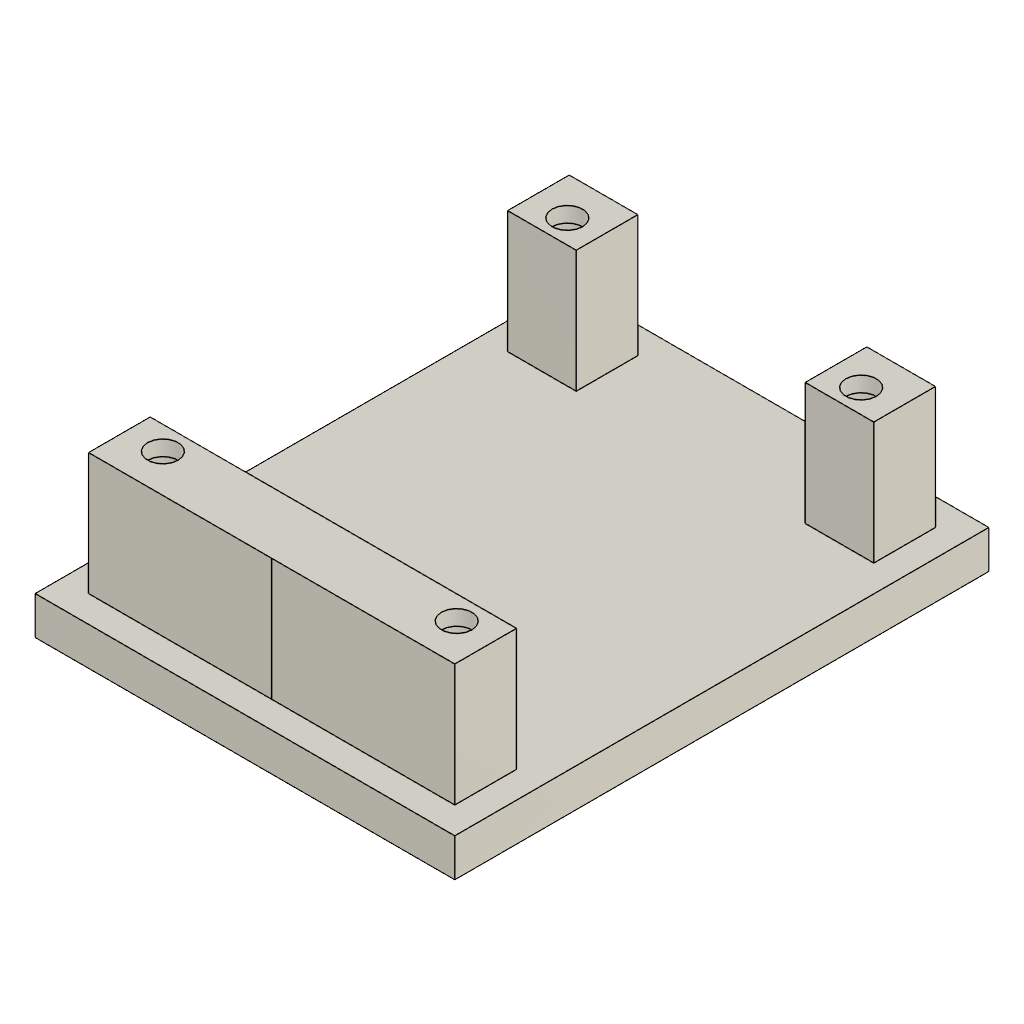
Case assembly (Autodesk Fusion 360 archive; units mm, degrees)
design "Board Case Top"
part number: 2026-09-13-14-46-25-976
Autodesk Fusion 360 part; units mm, degrees
sketch "Sketch1" plane through (0, 0, 0) normal (0, 0, 1) x (1, 0, 0)
  line L0 (25, 33) -> (-25, 33)
  line L1 (-27.5, 35) -> (-27.5, -35)
  line L2 (-25, 33) -> (-25, -33)
  line L3 (27.5, -35) -> (27.5, 35)
  circle A0 centre (19.25, -26.5) radius 2
  line L4 (-19.25, -26.5) -> (19.25, -26.5)
  line L5 (0, 0) -> (0, -26.5)
  circle A1 centre (19.25, 26.5) radius 2
  line L6 (0, 0) -> (0, 26.5)
  line L7 (27.5, 35) -> (-27.5, -35) construction
  circle A2 centre (-19.25, -26.5) radius 2
  line L8 (-25, 33) -> (25, -33) construction
  line L9 (25, 33) -> (-25, -33) construction
  line L10 (27.5, 35) -> (27.5, -35)
  line L11 (27.5, -35) -> (-27.5, -35)
  line L12 (27.5, 35) -> (-27.5, 35)
  line L13 (25, -33) -> (25, 33)
  line L14 (-27.5, -35) -> (-27.5, 35)
  line L15 (27.5, 35) -> (-27.5, 35)
  circle A3 centre (-19.25, 26.5) radius 2
  line L16 (-27.5, -35) -> (27.5, -35)
  line L17 (-27.5, 35) -> (27.5, -35) construction
  line L18 (-27.5, -35) -> (27.5, -35)
  line L19 (0, -35) -> (0, 35)
  line L20 (-19.25, 26.5) -> (19.25, 26.5)
  line L21 (-27.5, 35) -> (27.5, 35)
  line L22 (-25, -33) -> (25, -33)
  dimension "d2" = 70
  dimension "d3" = 55
  dimension "d4" = 55
  dimension "d5" = 26.5
  dimension "d6" = 26.5
  dimension "d7" = 38.5
  dimension "d8" = 38.5
  dimension "d9" = 4
  dimension "d10" = 4
  dimension "d11" = 4
  dimension "d12" = 4
  constraint midpoint L5.start L19
  constraint coincident L5.start L6.start
  constraint vertical L19
  constraint midpoint L19.end L15
  constraint perpendicular L15 L19
  constraint midpoint L19.start L16
  constraint perpendicular L16 L19
  constraint horizontal L21
  constraint vertical L10
  constraint horizontal L11
  constraint vertical L14
  constraint coincident L6.end L19
  constraint parallel L5 L19
  constraint midpoint L6.end L20
  constraint perpendicular L6 L20
  constraint midpoint L5.end L4
  constraint perpendicular L4 L19
  constraint coincident L4.start A2.centre
  constraint coincident A0.centre L4.end
  constraint coincident A1.centre L20.end
  constraint coincident A3.centre L20.start
  constraint horizontal L0
  constraint perpendicular L0 L2
  constraint parallel L0 L22
  constraint parallel L2 L13
  constraint coincident L5.start L9
  constraint coincident L5.start L8
  constraint horizontal L12
  constraint perpendicular L1 L12
  constraint parallel L12 L18
  constraint parallel L1 L3
  constraint coincident L5.start L7
  constraint coincident L5.start L17
  measures "d2" distance of L19.start L19.end
  measures "d3" distance of L3.end L1.start
  measures "d4" distance of L3.start L1.end
  measures "d5" distance of L6.end L5.start
  measures "d6" distance of L5.end L5.start
  measures "d7" distance of A3.centre A1.centre
  measures "d8" distance of A0.centre L4.start
  measures "d9" diameter of A2
  measures "d10" diameter of A0
  measures "d11" diameter of A1
  measures "d12" diameter of A3
extrude "Extrude1" add sketch "Sketch1" along normal blind 5
sketch "Sketch2" plane through (0, 0, 5) normal (0, 0, 1) x (-1, 0, 0)
  circle A0 centre (-19.25, 26.5) radius 2
  circle A1 centre (19.25, -26.5) radius 2
  circle A2 centre (19.25, 26.5) radius 2
  circle A3 centre (-19.25, -26.5) radius 2
  line L0 (27.5, 35) -> (-27.5, 35)
  line L1 (-27.5, 35) -> (-27.5, -35)
  line L2 (-27.5, -35) -> (27.5, -35)
  line L3 (27.5, -35) -> (27.5, 35)
  line L4 (19.25, -26.5) -> (-19.25, -26.5)
  line L5 (19.25, 26.5) -> (-19.25, 26.5)
  line L6 (-27.5, 29.5868) -> (27.5, 29.5868)
  line L7 (27.5, 29.5868) -> (27.5, 23.4132)
  line L8 (27.5, 23.4132) -> (-27.5, 23.4132)
  line L9 (-27.5, 23.4132) -> (-27.5, 29.5868)
  line L10 (-27.5, 29.5868) -> (27.5, 23.4132) construction
  line L11 (27.5, 29.5868) -> (-27.5, 23.4132) construction
  line L12 (-27.5, -29.5868) -> (-27.5, -23.4132)
  line L13 (-27.5, -23.4132) -> (27.5, -23.4132)
  line L14 (27.5, -29.5868) -> (-27.5, -29.5868)
  line L15 (27.5, -23.4132) -> (27.5, -29.5868)
  point P0 (0, 26.5)
  constraint coincident A1.centre L4.start
  constraint coincident A3.centre L4.end
  constraint coincident A2.centre L5.start
  constraint coincident A0.centre L5.end
  constraint horizontal L6
  constraint perpendicular L6 L7
  constraint parallel L6 L8
  constraint parallel L7 L9
  constraint coincident L10 P0
  constraint coincident L11 P0
  constraint coincident L1 L6.start
  constraint midpoint L5 P0
  constraint horizontal L13
  constraint perpendicular L13 L15
  constraint parallel L13 L14
  constraint parallel L12 L15
extrude "Extrude2" add sketch "Sketch2" along normal blind 16 contours L1 L3 L6 L7 L8 L9 | L1 L3 L12 L13 L14 L15
sketch "Sketch3" plane through (0, 0, 5) normal (0, 0, 1) x (-1, 0, 0)
  line L0 (27.5, 23.4132) -> (-27.5, 23.4132)
  line L1 (-27.5, 23.4132) -> (-27.5, -23.4132)
  line L2 (-27.5, -23.4132) -> (27.5, -23.4132)
  line L3 (27.5, -23.4132) -> (27.5, 23.4132)
  line L4 (-25, -32.5) -> (-25, 32.5)
  line L5 (-25, 32.5) -> (25, 32.5)
  line L6 (25, 32.5) -> (25, -32.5)
  line L7 (25, -32.5) -> (-25, -32.5)
  line L8 (25, -32.5) -> (-25, -32.5)
  line L9 (-25, -32.5) -> (-25, -29.5)
  line L10 (-25, -29.5) -> (25, -29.5)
  line L11 (25, -29.5) -> (25, -32.5)
  line L12 (25, 32.5) -> (-25, 32.5)
  line L13 (-25, 32.5) -> (-25, 29)
  line L14 (-25, 29) -> (25, 29)
  line L15 (25, 29) -> (25, 32.5)
  dimension "d17" = 65
  dimension "d18" = 50
  constraint horizontal L5
  constraint perpendicular L5 L6
  constraint parallel L5 L7
  constraint parallel L4 L6
  constraint horizontal L8
  constraint vertical L9
  constraint horizontal L10
  constraint vertical L11
  constraint coincident L4 L9.end
  constraint horizontal L12
  constraint vertical L13
  constraint horizontal L14
  constraint vertical L15
  constraint coincident L4 L13.end
  measures "d17" distance of L6.end L5.end
  measures "d18" distance of L6.end L4.start
extrude "Extrude3" add sketch "Sketch3" along normal blind 16 contours L4 L5 L6 L12 L13 L14 L15 | L4 L6 L7 L8 L9 L10 L11
sketch "Sketch4" plane through (0, 0, 5) normal (0, 0, 1) x (-1, 0, 0)
  line L0 (27.5, 23.4132) -> (-27.5, 23.4132)
  line L1 (-27.5, 23.4132) -> (-27.5, -23.4132)
  line L2 (-27.5, -23.4132) -> (27.5, -23.4132)
  line L3 (27.5, -23.4132) -> (27.5, 23.4132)
  line L4 (-25, -32.5) -> (-25, 32.5)
  line L5 (-25, 32.5) -> (25, 32.5)
  line L6 (25, 32.5) -> (25, -32.5)
  line L7 (25, -32.5) -> (-25, -32.5)
  line L8 (29, 36) -> (-29, 36)
  line L9 (-29, 36) -> (-29, -36)
  line L10 (-29, -36) -> (29, -36)
  line L11 (29, -36) -> (29, 36)
  line L12 (29, 36) -> (-29, -36) construction
  line L13 (-29, 36) -> (29, -36) construction
  dimension "d21" = 65
  dimension "d22" = 50
  constraint horizontal L5
  constraint perpendicular L5 L6
  constraint parallel L5 L7
  constraint parallel L4 L6
  constraint horizontal L8
  constraint perpendicular L8 L9
  constraint parallel L8 L10
  constraint parallel L9 L11
  constraint coincident L12 origin
  constraint coincident L13 origin
  measures "d21" distance of L6.end L5.end
  measures "d22" distance of L6.end L4.start
extrude "Extrude4" cut sketch "Sketch4" along normal blind 20
sketch "Sketch5" plane through (0, 0, 0) normal (0, 0, -1) x (1, 0, 0)
  circle A0 centre (19.25, 26.5) radius 2
  circle A1 centre (-19.25, -26.5) radius 2
  circle A2 centre (-19.25, 26.5) radius 2
  circle A3 centre (19.25, -26.5) radius 2
  line L0 (27.5, 35) -> (-27.5, 35)
  line L1 (-27.5, 35) -> (-27.5, -35)
  line L2 (-27.5, -35) -> (27.5, -35)
  line L3 (27.5, -35) -> (27.5, 35)
  circle A4 centre (19.25, -26.5) radius 3
  circle A5 centre (-19.25, -26.5) radius 3
  circle A6 centre (-19.25, 26.5) radius 3
  circle A7 centre (19.25, 26.5) radius 3
  dimension "d25" = 6
  dimension "d26" = 6
  dimension "d27" = 6
  dimension "d28" = 6
  constraint concentric A3 A4
  measures "d25" diameter of A4
  measures "d26" diameter of A5
  measures "d27" diameter of A6
  measures "d28" diameter of A7
extrude "Extrude5" cut sketch "Sketch5" against normal blind 19 contours A4 | A5 | A6 | A7
sketch "Sketch6" plane through (0, 0, 21) normal (0, 0, 1) x (-1, 0, 0)
  line L0 (-25, -23.4132) -> (-25, -32.5)
  line L1 (-25, -32.5) -> (25, -32.5)
  line L2 (25, -32.5) -> (25, -23.4132)
  line L3 (0, -32.5) -> (0, -31.5)
  line L4 (0, -31.5) -> (25, -31.5)
  line L5 (0, -31.5) -> (-24.1654, -31.5)
  line L6 (-24.1654, -31.5) -> (-25, -31.5)
  line L7 (-25, -31.5) -> (-25, -32.5)
  line L8 (-25, -32.5) -> (25, -32.5)
  line L9 (25, -32.5) -> (25, -31.5)
  line L10 (0, 0) -> (6, 0)
  line L11 (0, 31.5) -> (-24.1654, 31.5)
  line L12 (0, 31.5) -> (25, 31.5)
  line L13 (-25, 32.5) -> (25, 32.5)
  line L14 (25, 32.5) -> (25, 31.5)
  line L15 (-25, 31.5) -> (-25, 32.5)
  line L16 (-24.1654, 31.5) -> (-25, 31.5)
  line L17 (25, -23.4132) -> (-25, -23.4132)
  circle A0 centre (-19.25, -26.5) radius 2
  circle A1 centre (19.25, -26.5) radius 2
  dimension "d31" = 1
  constraint midpoint L1 L3.start
  constraint vertical L3
  constraint coincident L2 L4.end
  constraint perpendicular L2 L4
  constraint perpendicular L0 L5
  constraint coincident L0 L6.end
  constraint perpendicular L0 L6
  constraint coincident L0.end L1.start
  constraint coincident L1.end L2.start
  constraint coincident L10.start origin
  constraint horizontal L10
  constraint symmetric L3.end L10 L11.start
  constraint symmetric L4.end L10 L12.end
  constraint symmetric L5.end L10 L11.end
  constraint symmetric L6.end L10 L15.start
  constraint symmetric L0.end L10 L13.start
  constraint symmetric L1.end L10 L13.end
  measures "d31" distance of L3.start L3.end
extrude "Extrude6" cut sketch "Sketch6" against normal blind 16 contours L0 L1 L3 L5 L6 L7 L8 | L1 L2 L3 L4 L8 L9 | L11 L12 L13 L14 L15 L16
sketch "Sketch7" plane through (0, 0, 21) normal (0, 0, 1) x (-1, 0, 0)
  line L0 (0, -31.5) -> (25, -31.5)
  line L1 (25, -31.5) -> (25, -23.4132)
  line L2 (-25, -23.4132) -> (-25, -31.5)
  line L3 (-25, -31.5) -> (0, -31.5)
  line L4 (25, -27.4566) -> (24, -27.4566)
  line L5 (24, -27.4566) -> (24, -31.5)
  line L6 (24, -27.4566) -> (24, -23.4132)
  line L7 (24, -23.4132) -> (25, -23.4132)
  line L8 (25, -31.5) -> (25, -23.4132)
  line L9 (25, -31.5) -> (24, -31.5)
  line L10 (0, -31.5) -> (0, -23.4132)
  line L11 (-25, -31.5) -> (-25, -23.4132)
  line L12 (-24, -27.4566) -> (-24, -23.4132)
  line L13 (-24, -27.4566) -> (-24, -31.5)
  line L14 (-25, -31.5) -> (-24, -31.5)
  line L15 (-24, -23.4132) -> (-25, -23.4132)
  line L16 (6, 0) -> (-5, 0)
  line L17 (24, 27.4566) -> (24, 23.4132)
  line L18 (24, 27.4566) -> (24, 31.5)
  line L19 (25, 31.5) -> (25, 23.4132)
  line L20 (25, 31.5) -> (24, 31.5)
  line L21 (24, 23.4132) -> (25, 23.4132)
  line L22 (-24, 27.4566) -> (-24, 31.5)
  line L23 (-24, 27.4566) -> (-24, 23.4132)
  line L24 (-25, 31.5) -> (-25, 23.4132)
  line L25 (-25, 31.5) -> (-24, 31.5)
  line L26 (-24, 23.4132) -> (-25, 23.4132)
  circle A0 centre (19.25, -26.5) radius 2
  circle A1 centre (-19.25, -26.5) radius 2
  line L27 (25, -23.4132) -> (-25, -23.4132)
  constraint midpoint L1 L4.start
  constraint perpendicular L1 L4
  constraint coincident L0 L5.end
  constraint perpendicular L0 L5
  constraint coincident L1.end L7.end
  constraint coincident L0.end L1.start
  constraint coincident L0.start L3.end
  constraint symmetric L4.end L10 L12.start
  constraint symmetric L5.end L10 L13.end
  constraint symmetric L6.end L10 L12.end
  constraint symmetric L1.end L10 L2.start
  constraint symmetric L0.end L10 L2.end
  constraint horizontal L16
  constraint symmetric L4.end L16 L17.start
  constraint symmetric L5.end L16 L18.end
  constraint symmetric L6.end L16 L17.end
  constraint symmetric L1.end L16 L19.end
  constraint symmetric L0.end L16 L19.start
  constraint symmetric L2.end L16 L24.start
  constraint symmetric L2.start L16 L24.end
  constraint symmetric L12.start L16 L22.start
  constraint symmetric L12.end L16 L23.end
  constraint symmetric L13.end L16 L22.end
extrude "Extrude7" cut sketch "Sketch7" against normal blind 16 contours L0 L1 L4 L5 L8 L9 | L2 L3 L11 L12 L13 L14 L15 L27 | L1 L4 L6 L7 L8 L27 | L17 L18 L19 L20 L21 | L22 L23 L24 L25 L26
sketch "Sketch8" plane through (0, 23.4132, 0) normal (0, -1, 0) x (1, 0, 0)
  line L0 (24, 5) -> (24, 21)
  line L1 (24, 21) -> (-24, 21)
  line L2 (-24, 21) -> (-24, 5)
  line L3 (-24, 5) -> (24, 5)
  line L4 (-15, 21) -> (15, 21)
  line L5 (15, 21) -> (15, 5)
  line L6 (15, 5) -> (-15, 5)
  line L7 (-15, 5) -> (-15, 21)
  constraint horizontal L4
  constraint vertical L5
  constraint horizontal L6
  constraint vertical L7
  constraint coincident L1 L4.start
extrude "Extrude8" cut sketch "Sketch8" against normal blind 23 contours L1 L3 L4 L5 L6 L7

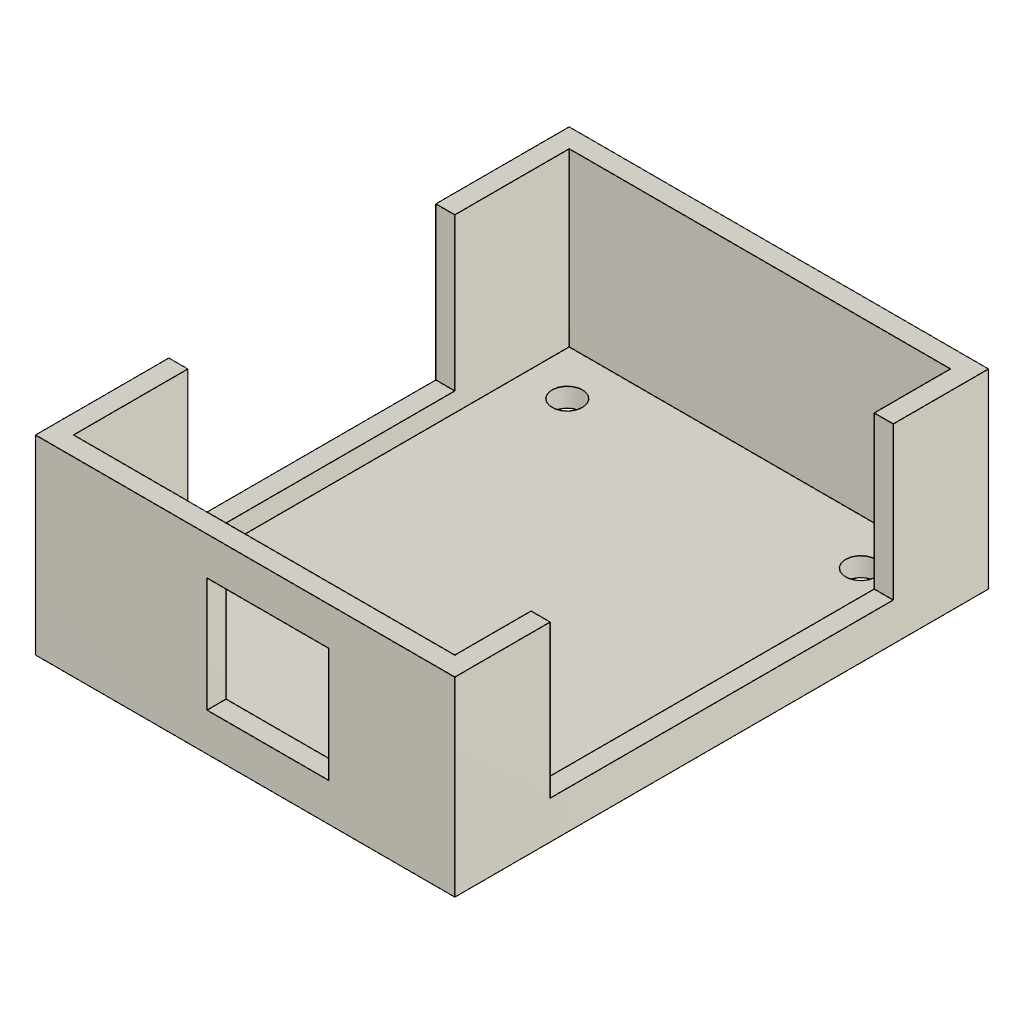
design "Board Case Bottem"
part number: 2026-09-12-19-48-28-623
Autodesk Fusion 360 part; units mm, degrees
sketch "Sketch1" plane through (0, 0, 0) normal (0, 0, 1) x (1, 0, 0)
  line L0 (0, -35) -> (0, 35)
  line L1 (27.5, 35) -> (-27.5, 35)
  line L2 (-27.5, -35) -> (27.5, -35)
  line L3 (-27.5, 35) -> (27.5, 35)
  line L4 (27.5, 35) -> (27.5, -35)
  line L5 (27.5, -35) -> (-27.5, -35)
  line L6 (-27.5, -35) -> (-27.5, 35)
  line L7 (0, 0) -> (0, 26.5)
  line L8 (0, 0) -> (0, -26.5)
  line L9 (-19.25, 26.5) -> (19.25, 26.5)
  line L10 (-19.25, -26.5) -> (19.25, -26.5)
  circle A0 centre (-19.25, -26.5) radius 2
  circle A1 centre (19.25, -26.5) radius 2
  circle A2 centre (19.25, 26.5) radius 2
  circle A3 centre (-19.25, 26.5) radius 2
  line L11 (25, 33) -> (-25, 33)
  line L12 (-25, 33) -> (-25, -33)
  line L13 (-25, -33) -> (25, -33)
  line L14 (25, -33) -> (25, 33)
  line L15 (25, 33) -> (-25, -33) construction
  line L16 (-25, 33) -> (25, -33) construction
  line L17 (27.5, 35) -> (-27.5, 35)
  line L18 (-27.5, 35) -> (-27.5, -35)
  line L19 (-27.5, -35) -> (27.5, -35)
  line L20 (27.5, -35) -> (27.5, 35)
  line L21 (27.5, 35) -> (-27.5, -35) construction
  line L22 (-27.5, 35) -> (27.5, -35) construction
  dimension "d1" = 70
  dimension "d2" = 55
  dimension "d3" = 55
  dimension "d4" = 26.5
  dimension "d5" = 26.5
  dimension "d6" = 38.5
  dimension "d7" = 38.5
  dimension "d8" = 4
  dimension "d9" = 4
  dimension "d10" = 4
  dimension "d11" = 4
  constraint midpoint L0 L7.start
  constraint coincident L7.start L8.start
  constraint vertical L0
  constraint midpoint L0.end L1
  constraint perpendicular L0 L1
  constraint midpoint L0.start L2
  constraint perpendicular L0 L2
  constraint horizontal L3
  constraint vertical L4
  constraint horizontal L5
  constraint vertical L6
  constraint coincident L0 L7.end
  constraint parallel L0 L8
  constraint midpoint L7.end L9
  constraint perpendicular L7 L9
  constraint midpoint L8.end L10
  constraint perpendicular L0 L10
  constraint coincident L10.start A0.centre
  constraint coincident L10.end A1.centre
  constraint coincident L9.end A2.centre
  constraint coincident L9.start A3.centre
  constraint horizontal L11
  constraint perpendicular L11 L12
  constraint parallel L11 L13
  constraint parallel L12 L14
  constraint coincident L15 L7.start
  constraint coincident L16 L7.start
  constraint horizontal L17
  constraint perpendicular L17 L18
  constraint parallel L17 L19
  constraint parallel L18 L20
  constraint coincident L21 L7.start
  constraint coincident L22 L7.start
  measures "d1" distance of L0.start L0.end
  measures "d2" distance of L1.start L1.end
  measures "d3" distance of L2.start L2.end
  measures "d4" distance of L7.start L7.end
  measures "d5" distance of L7.start L8.end
  measures "d6" distance of L9.start L9.end
  measures "d7" distance of L10.start L10.end
  measures "d8" diameter of A0
  measures "d9" diameter of A1
  measures "d10" diameter of A2
  measures "d11" diameter of A3
extrude "Extrude1" add sketch "Sketch1" along normal blind 5
sketch "Sketch2" plane through (0, 0, 5) normal (0, 0, 1) x (-1, 0, 0)
  circle A0 centre (-19.25, -26.5) radius 2
  circle A1 centre (19.25, -26.5) radius 2
  circle A2 centre (-19.25, 26.5) radius 2
  circle A3 centre (19.25, 26.5) radius 2
  line L0 (-27.5, 35) -> (-27.5, -35)
  line L1 (-27.5, -35) -> (27.5, -35)
  line L2 (27.5, -35) -> (27.5, 35)
  line L3 (27.5, 35) -> (-27.5, 35)
  line L4 (-27.5, -35) -> (27.5, -35)
  line L5 (27.5, -35) -> (27.5, 35)
  line L6 (27.5, 35) -> (-27.5, 35)
  line L7 (-27.5, 35) -> (-27.5, -35)
  line L8 (-27.5, -35) -> (27.5, 35) construction
  line L9 (27.5, -35) -> (-27.5, 35) construction
  line L10 (-25, 32.5) -> (25, 32.5)
  line L11 (25, 32.5) -> (25, -32.5)
  line L12 (25, -32.5) -> (-25, -32.5)
  line L13 (-25, -32.5) -> (-25, 32.5)
  line L14 (-25, 32.5) -> (25, -32.5) construction
  line L15 (25, 32.5) -> (-25, -32.5) construction
  dimension "d14" = 65
  dimension "d15" = 50
  constraint horizontal L4
  constraint perpendicular L4 L5
  constraint parallel L4 L6
  constraint parallel L5 L7
  constraint coincident L8 origin
  constraint coincident L9 origin
  constraint coincident L0.end L1.start
  constraint horizontal L10
  constraint perpendicular L10 L11
  constraint parallel L10 L12
  constraint parallel L11 L13
  constraint coincident L14 origin
  constraint coincident L15 origin
  measures "d14" distance of L10.end L11.end
  measures "d15" distance of L11.end L12.end
extrude "Extrude2" add sketch "Sketch2" along normal blind 20 contours L0 L1 L2 L3 L4 L5 L6 L7
sketch "Sketch3" plane through (-27.5, 0, 0) normal (-1, 0, 0) x (0, -1, 0)
  line L0 (-35, 0) -> (35, 0)
  line L1 (35, 0) -> (35, 25)
  line L2 (35, 25) -> (-35, 25)
  line L3 (-35, 25) -> (-35, 0)
  line L4 (0, 0) -> (0, 5)
  line L5 (-17.5, 5) -> (17.5, 5)
  line L6 (-17.5, 5) -> (-17.5, 25)
  line L7 (17.5, 5) -> (17.5, 25)
  line L8 (-17.5, 25) -> (17.5, 25)
  dimension "d18" = 5
  dimension "d19" = 35
  constraint coincident L4.start origin
  constraint perpendicular L0 L4
  constraint midpoint L4.end L5
  constraint perpendicular L4 L5
  constraint coincident L2 L6.end
  constraint perpendicular L2 L6
  constraint coincident L2 L7.end
  constraint perpendicular L2 L7
  measures "d18" distance of L4.start L4.end
  measures "d19" distance of L5.start L5.end
extrude "Extrude3" cut sketch "Sketch3" against normal blind 20 contours L2 L5 L6 L7 L8
sketch "Sketch4" plane through (25, 0, 0) normal (-1, 0, 0) x (0, -1, 0)
  line L0 (-32.5, 5) -> (32.5, 5)
  line L1 (32.5, 5) -> (32.5, 25)
  line L2 (32.5, 25) -> (-32.5, 25)
  line L3 (-32.5, 25) -> (-32.5, 5)
  line L4 (0, 0) -> (0, 5)
  line L5 (22.5, 5) -> (-22.5, 5)
  line L6 (-22.5, 5) -> (-22.5, 25)
  line L7 (22.5, 5) -> (22.5, 25)
  line L8 (22.5, 25) -> (-22.5, 25)
  dimension "d22" = 45
  constraint coincident L4.start origin
  constraint midpoint L0 L4.end
  constraint midpoint L4.end L5
  constraint perpendicular L4 L5
  constraint coincident L2 L6.end
  constraint perpendicular L2 L6
  constraint perpendicular L5 L7
  constraint perpendicular L6 L8
  measures "d22" distance of L5.start L5.end
extrude "Extrude4" cut sketch "Sketch4" against normal blind 51 contours L0 L2 L5 L6 L7 L8
sketch "Sketch5" plane through (0, 0, 5) normal (0, 0, 1) x (-1, 0, 0)
  circle A0 centre (19.25, 26.5) radius 2
  circle A1 centre (-19.25, 26.5) radius 2
  circle A2 centre (19.25, -26.5) radius 2
  circle A3 centre (-19.25, -26.5) radius 2
  line L0 (25, 17.5) -> (25, 32.5)
  line L1 (25, 32.5) -> (-25, 32.5)
  line L2 (-25, 32.5) -> (-25, 22.5)
  line L3 (-25, 22.5) -> (-27.5, 22.5)
  line L4 (-27.5, 22.5) -> (-27.5, -22.5)
  line L5 (-27.5, -22.5) -> (-25, -22.5)
  line L6 (-25, -22.5) -> (-25, -32.5)
  line L7 (-25, -32.5) -> (25, -32.5)
  line L8 (25, -32.5) -> (25, -17.5)
  line L9 (25, -17.5) -> (27.5, -17.5)
  line L10 (27.5, -17.5) -> (27.5, 17.5)
  line L11 (27.5, 17.5) -> (25, 17.5)
  line L12 (-25, 32.5) -> (25, 32.5)
  line L13 (25, 32.5) -> (25, -32.5)
  line L14 (25, -32.5) -> (-25, -32.5)
  line L15 (-25, -32.5) -> (-25, 32.5)
  constraint horizontal L12
  constraint vertical L13
  constraint horizontal L14
  constraint vertical L15
  constraint coincident L7.end L8.start
  constraint coincident L1.end L2.start
extrude "Extrude5" cut sketch "Sketch5" against normal blind 2.5 contours L0 L1 L2 L6 L7 L8 L12 L13 L14 L15
sketch "Sketch7" plane through (0, -32.5, 0) normal (0, 1, 0) x (-1, 0, 0)
  line L0 (25, 2.5) -> (25, 25)
  line L1 (25, 25) -> (-25, 25)
  line L2 (-25, 25) -> (-25, 2.5)
  line L3 (-25, 2.5) -> (25, 2.5)
  line L4 (-10.9638, 20) -> (5, 20)
  line L5 (5, 20) -> (5, 5)
  line L6 (5, 5) -> (-10.9638, 5)
  line L7 (-10.9638, 5) -> (-10.9638, 20)
  constraint horizontal L4
  constraint vertical L5
  constraint horizontal L6
  constraint vertical L7
extrude "Extrude7" cut sketch "Sketch7" against normal blind 8 contours L4 L5 L6 L7
